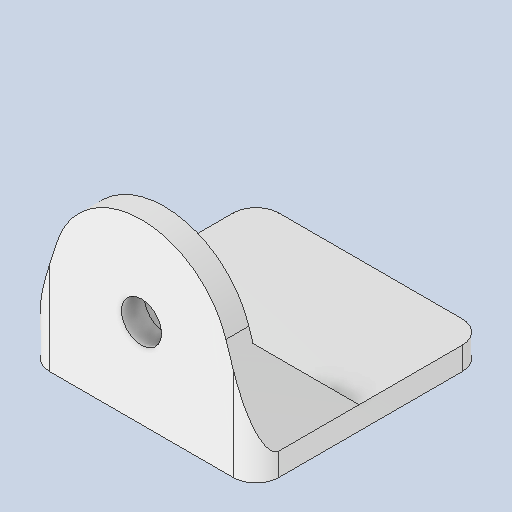
# Autodesk Inventor part: ChargingArm - FlatPlateBracket
Saved by Autodesk Inventor 2023 (Build 270158000, 158)
## iProperties
Created: 2023-04-05
Part Number: ChargingArm - FlatPlateBracket
Material: ABS Plastic
Document SubType Name: Modeling
Designer: Administrator
Density: 1.06 g/cm^3
Appearance: Smooth - White
Author: Administrator
Autodesk Inventor part; units mm, degrees
ref_plane "YZ Plane" through (0, 0, 0) normal (1, 0, 0) x (0, 1, 0)
ref_plane "XZ Plane" through (0, 0, 0) normal (0, 1, 0) x (-1, 0, 0)
ref_plane "XY Plane" through (0, 0, 0) normal (0, 0, 1) x (1, 0, 0)
sketch "Sketch1" plane through (0, 0, 0) normal (1, 0, 0) x (0, 1, 0)
  line L0 (0, 0) -> (20, 0)
  line L1 (20, 0) -> (20, -20)
  line L2 (20, -20) -> (0, -20)
  line L3 (0, -20) -> (0, 0)
  dimension "d0" = 20
  dimension "d1" = 20
  constraints: 8 end point, 2 parallel, 1 horizontal, 1 perpendicular
  measures "d0" distance of L1.end L2.end
  measures "d1" distance of L0.end L1.end
extrude "Extrusion1" add sketch "Sketch1" along normal blind 2
sketch "Sketch3" plane through (0, 20, 0) normal (0, 1, 0) x (1, 0, 0)
  circle A0 centre (7.75, 10) radius 7.75
  line L0 (2, 20) -> (2, 0) projected
  line L1 (2, 0) -> (10.1308, 2.6248)
  line L2 (2, 20) -> (10.1308, 17.3752)
  circle A1 centre (7.75, 10) radius 1.75
  line L3 (0, 20) -> (0, 0) projected
  dimension "d11" = 15.5
  dimension "d12" = 3.5
  constraints: 4 end point, 3 tangent, 2 centre point, 2 point on circle, 1 coincident, 1 equal length
  measures "d11" diameter of A0
  measures "d12" diameter of A1
extrude "Extrusion3" add sketch "Sketch3" against normal blind 2 contours A0 L0 | A0 L0 L2 | L1 L0 A0 picked at (3.3333, 10)
chamfer "Chamfer3" distance 7 angle 45 1 edges at (2, 18, -10)
fillet "Fillet1" radius 2 4 edges at (1, 20, 0) (1, 0, 0) (1, 20, -20) (1, 0, -20)
sketch "Sketch4" plane through (0, 18, 0) normal (0, -1, 0) x (1, 0, 0)
  arc A0 (9, -11.2247) -> (9, -8.7753) centre (7.75, -10) ccw projected
  circle A1 centre (7.75, -10) radius 4.5
  point P0 (0, 0)
  dimension "d22" = 9
  constraints: 1 centre point, 1 coincident
  measures "d22" diameter of A1
extrude "Extrusion4" cut sketch "Sketch4" along normal blind 6
body "Solid1"
